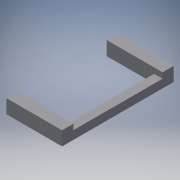
# Autodesk Inventor part: emmerhouder
Saved by Autodesk Inventor 2017 (Build 210142000, 142)
## iProperties
Created: 2017-02-19
Part Number: emmerhouder
Material: Generic
Document SubType Name: Modeling
Designer: user
Density: 1 g/cm^3
Appearance: Default
Author: user
Autodesk Inventor part; units mm, degrees
ref_plane "YZ Plane" through (0, 0, 0) normal (1, 0, 0) x (0, 1, 0)
ref_plane "XZ Plane" through (0, 0, 0) normal (0, 1, 0) x (-1, 0, 0)
ref_plane "XY Plane" through (0, 0, 0) normal (0, 0, 1) x (1, 0, 0)
sketch "Sketch1" plane through (0, 0, 0) normal (0, 0, 1) x (1, 0, 0)
  line L0 (40, 160) -> (876.7461, 160) projected
  line L1 (876.7461, 160) -> (876.7461, -160) projected
  line L2 (876.7461, -160) -> (40, -160) projected
  line L3 (40, -200) -> (40, -160) projected
  line L4 (916.7461, -200) -> (40, -200) projected
  line L5 (916.7461, -160) -> (916.7461, -200) projected
  line L6 (916.7461, 160) -> (916.7461, -160) projected
  line L7 (916.7461, 200) -> (916.7461, 160) projected
  line L8 (40, 200) -> (916.7461, 200) projected
  line L9 (40, 160) -> (40, 200) projected
  line L10 (618.4585, 200) -> (418.4585, 200)
  line L11 (418.4585, 200) -> (418.4585, 160)
  line L12 (418.4585, 160) -> (618.4585, 160)
  line L13 (618.4585, 160) -> (618.4585, 200)
  line L14 (618.4585, -160) -> (418.4585, -160)
  line L15 (418.4585, -160) -> (418.4585, -200)
  line L16 (418.4585, -200) -> (618.4585, -200)
  line L17 (618.4585, -200) -> (618.4585, -160)
  point P0 (0, 0)
  dimension "d0" = 200
  constraints: 16 end point, 6 point on line, 4 parallel, 2 horizontal, 2 perpendicular
  measures "d0" distance between parallel lines of L15 L17
extrude "Extrusion1" add sketch "Sketch1" along normal blind 50 contours L11 L8 L13 L0 | L17 L4 L15 L2
sketch "Sketch2" plane through (418.4585, -160, 0) normal (0, 1, 0) x (1, 0, 0)
  arc A0 (78.7868, -178.7868) -> (121.2132, -178.7868) centre (100, -157.5736) ccw projected
  arc A1 (78.7868, -178.7868) -> (121.2132, -178.7868) centre (100, -157.5736) ccw projected
  circle A2 centre (100, -157.5736) radius 10
  line L0 (0, 0) -> (0, -50) projected
  line L1 (0, 0) -> (200, 0) projected
  line L2 (200, 0) -> (200, -50) projected
  line L3 (200, 0) -> (200, -87.5736) projected
  line L4 (200, 0) -> (170, 0)
  line L5 (170, 0) -> (170, -30)
  line L6 (170, -30) -> (200, -30)
  line L7 (200, -30) -> (200, 0)
  line L8 (0, -50) -> (200, -50) projected
  point P0 (-418.4585, 0)
  dimension "d7" = 20
  dimension "d10" = 30
  dimension "d11" = 30
  constraints: 8 end point, 2 parallel, 1 centre point, 1 coincident, 1 horizontal, 1 perpendicular
  measures "d7" diameter of A2
  measures "d10" distance of L4.end L5.end
  measures "d11" distance of L5.end L6.end
extrude "Extrusion2" add sketch "Sketch2" along normal up to next contours L1 L2 L6 L5
sketch "Sketch3" plane through (618.4585, -200, 0) normal (1, 0, 0) x (0, 0, -1)
  line L0 (-30, 40) -> (-30, 360) projected
  line L1 (-30, 40) -> (-50, 40) projected
  line L2 (-50, 0) -> (-50, 40) projected
  line L3 (0, 0) -> (-50, 0) projected
  line L4 (0, 0) -> (0, 400) projected
  line L5 (0, 400) -> (-50, 400) projected
  line L6 (-50, 360) -> (-50, 400) projected
  line L7 (-30, 360) -> (-50, 360) projected
  line L8 (-30, 40) -> (-30, 360) projected
  line L9 (-30, 305) -> (-150, 305)
  arc A0 (-150, 305) -> (-150, 95) centre (-150, 200) ccw
  line L10 (-150, 95) -> (-30, 95)
  line L11 (-30, 305) -> (-30, 95)
  circle A1 centre (-150, 200) radius 85
  point P0 (0, 200)
  point P1 (0, 200)
  dimension "d13" = 170
  dimension "d14" = 20
  dimension "d15" = 120
  constraints: 6 end point, 2 centre point, 2 perpendicular, 2 point on circle, 2 point on line, 2 tangent, 1 coincident, 1 horizontal, 1 horizontal alignment, 1 midpoint
  measures "d13" diameter of A1
  measures "d14" radial gap between concentric circles of A0 A1
  measures "d15" distance from line of L0 A1.centre
extrude "Extrusion3" add sketch "Sketch3" against normal blind 30 contours L10 A0 L9 L0
body "Solid1"
